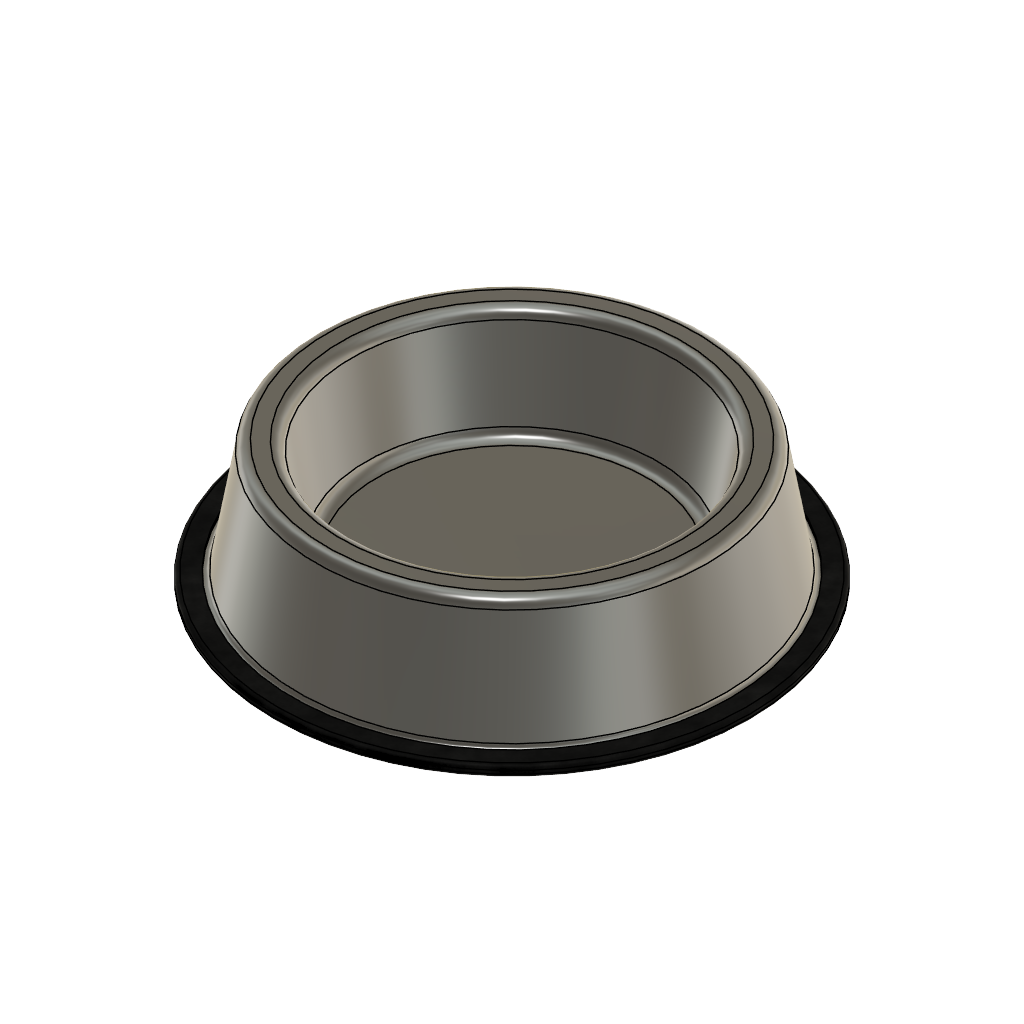
Dog Bowl (Autodesk Fusion 360 design; units mm, degrees)
part number: 2026-09-16-15-58-01-810
Autodesk Fusion 360 part; units mm, degrees
sketch "Sketch1" plane through (0, 0, 0) normal (0, 1, 0) x (1, 0, 0)
  line L0 (0, 0) -> (110, 0) construction
  line L1 (110, 0) -> (110, -2.5)
  line L2 (110, -2.5) -> (100, -2.5)
  line L3 (100, -2.5) -> (90.4494, -56.6644)
  line L4 (100, -2.5) -> (109.8395, -2.5) construction
  line L5 (90.4494, -56.6644) -> (75.4494, -56.6644)
  line L6 (75.4494, -56.6644) -> (67.2212, -10)
  line L7 (0, -10) -> (67.2212, -10)
  dimension "d17" = 110
  dimension "d18" = 2.5
  dimension "d19" = 10
  dimension "d20" = 100
  dimension "d21" = 55
  dimension "d22" = 15
  dimension "d23" = 10
  dimension "d24" = 100
  constraint coincident L0.start origin
  constraint horizontal L0
  constraint perpendicular L0 L1
  constraint perpendicular L1 L2
  constraint horizontal L4
  constraint horizontal L5
  constraint parallel L0 L7
  constraint vertical L0.start L7.start
  measures "d17" distance of L0.start L0.end
  measures "d18" distance of L0.end L1.end
  measures "d19" distance of L1.end L2.end
  measures "d20" angle of L3 L4
  measures "d21" distance of L2.end L3.end
  measures "d22" distance of L3.end L5.end
  measures "d23" distance of L0 L7
  measures "d24" angle of L6 L7
surface "Revolve2" add revolved angle 360 about axis through (0, 0, 1.75) along (0, 0, 20.75) path "Sketch1" along L1 L2 L3 L5 L6 L7 makes body 1
fillet "Fillet2" radius 5 3 edges at (-84.3284, -32.7079, 56.6644) (-70.3435, -27.2836, 56.6644) (-62.6721, -24.3082, 10) on bodies 1
fillet "Fillet2" radius 2.5 1 edges at (-93.2327, -36.1615, 2.5) on bodies 1
thicken "Thicken1" add thickness -2.5 9 faces at (95.7351, 14.4297, 20.5548) (-15.4183, 87.4414, 55.9733) (83.7297, -4.2852, 56.6644) (67.7617, 41.4083, 56.659) (16.1247, -70.647, 39.7324) (65.6103, 16.7064, 13.2353) (10.0484, 37.9024, 10) (-76.4529, 64.1516, 4.0098) (106.9564, -5.4649, 2.5) separate body on bodies 1 makes body 2
fillet "Fillet3" radius 0.5 2 edges at (-102.556, -39.7777, 2.5) (-102.556, -39.7777, 0) on bodies 2
offset_surface "SurfaceOffset1" offset 0.3 5 faces at (87.6312, 66.378, 0.25) (19.1013, -108.3289, 1) (-13.6695, -109.0798, 2.25) (106.6249, -5.44, 2.5) (106.6249, -5.44, 0) on bodies 2 makes body 3
thicken "Thicken2" add thickness 1 5 faces at (106.6249, -5.44, 2.8) (50.2711, -98.0575, 2.4) (-29.8737, -106.1775, 1) (87.8383, 66.5349, 0.1) (106.6249, -5.44, -0.3) separate body on bodies 3 makes body 4
